Autodesk Fusion 360 part; units mm, degrees
(part 2 of 3)
sketch "Arduino" plane through (0, 0, 0) normal (0, 0, 1) x (1, 0, 0)
  line L0 (-12.271, 37.48) -> (-12.271, 41.88)
  line L1 (-4.5943, 42.08) -> (-4.7943, 41.88)
  line L2 (0, 0) -> (0, 43.18)
  line L3 (-4.7943, 42.88) -> (-4.5943, 42.68)
  line L4 (-6.271, 42.88) -> (-4.7943, 42.88)
  line L5 (-6.271, 36.18) -> (-12.271, 36.18)
  line L6 (0, 43.18) -> (-6.271, 43.18)
  line L7 (-12.271, 41.88) -> (-13.7477, 41.88)
  line L8 (-13.9477, 42.68) -> (-13.7477, 42.88)
  line L9 (-11.771, 0) -> (-6.771, 0)
  arc A0 (-4.5943, 37.28) -> (-4.5943, 36.68) centre (-4.2943, 36.98) ccw
  arc A1 (-13.9477, 42.08) -> (-13.9477, 42.68) centre (-14.2477, 42.38) ccw
  line L10 (-18.542, 43.18) -> (-18.542, 0)
  line L11 (-12.271, 36.18) -> (-12.271, 36.48)
  line L12 (-6.771, 0) -> (0, 0)
  arc A2 (-13.7477, 42.88) -> (-12.271, 42.88) centre (-13.0093, 43.6183) ccw
  arc A3 (-4.5943, 42.68) -> (-4.5943, 42.08) centre (-4.2943, 42.38) ccw
  arc A4 (-13.7477, 37.48) -> (-12.271, 37.48) centre (-13.0093, 38.2183) ccw
  arc A5 (-13.9477, 36.68) -> (-13.9477, 37.28) centre (-14.2477, 36.98) ccw
  line L13 (-18.542, 43.18) -> (0, 43.18)
  line L14 (-6.271, 41.88) -> (-6.271, 37.48)
  line L15 (-6.271, 43.18) -> (-6.271, 42.88)
  line L16 (-18.542, 0) -> (-11.771, 0)
  line L17 (-6.271, 37.48) -> (-4.7943, 37.48)
  arc A6 (-4.7943, 36.48) -> (-6.271, 36.48) centre (-5.5326, 35.7416) ccw
  line L18 (-6.271, 36.48) -> (-6.271, 36.18)
  line L19 (-4.7943, 37.48) -> (-4.5943, 37.28)
  line L20 (-4.5943, 36.68) -> (-4.7943, 36.48)
  line L21 (-13.9477, 37.28) -> (-13.7477, 37.48)
  line L22 (-13.7477, 41.88) -> (-13.9477, 42.08)
  line L23 (-12.2841, 24.6374) -> (-12.2912, 24.6445)
  line L24 (-7.771, 0.9965) -> (-6.511, 0.9965)
  circle A7 centre (-17.018, 19.156) radius 0.5
  line L25 (-12.4229, 30.5196) -> (-12.8135, 30.9102)
  circle A8 centre (-17.018, 11.656) radius 0.5
  arc A9 (-4.7943, 41.88) -> (-6.271, 41.88) centre (-5.5326, 41.1416) ccw
  circle A10 centre (-17.018, 4.156) radius 0.5
  line L26 (-8.3809, 32.7815) -> (-8.7353, 33.1359)
  line L27 (-1.524, 19.156) -> (-1.024, 19.156)
  line L28 (-5.671, 30.8528) -> (-6.0616, 30.4622)
  line L29 (-7.271, 0.2361) -> (-7.271, 1.7561)
  line L30 (-6.0786, 0) -> (-12.4635, 0)
  line L31 (-11.771, 13.9686) -> (-11.771, 18.0694)
  circle A11 centre (-17.018, 14.156) radius 0.5
  circle A12 centre (-1.524, 9.156) radius 0.5
  line L32 (-6.3515, 30.7521) -> (-5.9609, 31.1427)
  circle A13 centre (-1.524, 11.656) radius 0.5
  line L33 (-12.271, 42.88) -> (-12.271, 43.18)
  line L34 (-12.5236, 31.2001) -> (-12.133, 30.8096)
  circle A14 centre (-1.524, 19.156) radius 0.5
  circle A15 centre (-17.018, 6.656) radius 0.889
  line L35 (-6.0616, 30.4622) -> (-6.3515, 30.7521)
  arc A16 (-5.671, 31.1356) -> (-5.671, 30.8528) centre (-5.8124, 30.9942) cw
  circle A17 centre (-7.271, 3.0017) radius 0.76
  line L36 (-8.0618, 33.5265) -> (-7.9903, 33.4549)
  arc A18 (-12.0012, 24.6374) -> (-12.2841, 24.6374) centre (-12.1427, 24.7789) cw
  circle A19 centre (-17.018, 9.156) radius 0.5
  circle A20 centre (-1.524, 14.156) radius 0.5
  line L37 (-11.6107, 25.028) -> (-12.0012, 24.6374)
  line L38 (-1.524, 24.156) -> (-1.024, 24.156)
  circle A21 centre (-17.018, 9.156) radius 0.889
  line L39 (-12.4635, 4.2) -> (-6.0786, 4.2)
  line L40 (-12.271, 36.48) -> (-13.7477, 36.48)
  line L41 (-1.524, 21.656) -> (-1.024, 21.656)
  line L42 (-8.7353, 33.1359) -> (-8.3447, 33.5265)
  arc A22 (-5.9609, 31.1427) -> (-5.6781, 31.1427) centre (-5.8195, 31.0013) cw
  circle A23 centre (-1.524, 16.656) radius 0.889
  line L43 (-11.9006, 25.3179) -> (-11.6107, 25.028)
  line L44 (-7.9903, 33.1721) -> (-8.3809, 32.7815)
  line L45 (-12.271, 43.18) -> (-18.542, 43.18)
  line L46 (-12.8135, 31.1931) -> (-12.8065, 31.2001)
  arc A24 (-12.8065, 31.2001) -> (-12.5236, 31.2001) centre (-12.665, 31.0587) cw
  line L47 (-12.4635, 0) -> (-12.4635, 4.2)
  circle A25 centre (-1.524, 9.156) radius 0.889
  line L48 (-17.018, 12.156) -> (-17.018, 11.156)
  circle A26 centre (-17.018, 11.656) radius 0.889
  line L49 (-11.771, 18.0694) -> (-6.771, 18.0694)
  line L50 (-6.0786, 4.2) -> (-6.0786, 0)
  circle A27 centre (-1.524, 6.656) radius 0.889
  line L51 (0, 43.18) -> (-18.542, 43.18)
  circle A28 centre (-1.524, 16.656) radius 0.5
  circle A29 centre (-17.018, 19.156) radius 0.889
  circle A30 centre (-17.018, 14.156) radius 0.889
  line L52 (-13.7477, 36.48) -> (-13.9477, 36.68)
  circle A31 centre (-1.524, 24.156) radius 0.889
  arc A32 (-12.8135, 30.9102) -> (-12.8135, 31.1931) centre (-12.6721, 31.0517) cw
  line L53 (-12.133, 30.8096) -> (-12.4229, 30.5196)
  line L54 (-16.518, 19.156) -> (-17.018, 19.156)
  circle A33 centre (-1.524, 14.156) radius 0.889
  line L55 (-12.2912, 24.9274) -> (-11.9006, 25.3179)
  circle A34 centre (-17.018, 16.656) radius 0.889
  circle A35 centre (-1.524, 24.156) radius 0.5
  circle A36 centre (-9.271, 3) radius 0.76
  arc A37 (-7.9903, 33.4549) -> (-7.9903, 33.1721) centre (-8.1317, 33.3135) cw
  line L56 (-1.524, 39.156) -> (-1.024, 39.156)
  line L57 (-14.0003, 28.4507) -> (-9.5417, 32.9093)
  line L58 (-9.0003, 32.9093) -> (-4.5417, 28.4507)
  line L59 (-14.0589, 28.0507) -> (-14.0589, 28.3093)
  circle A38 centre (-1.524, 4.156) radius 0.889
  line L60 (-17.518, 11.656) -> (-16.518, 11.656)
  arc A39 (-6.5407, 31.7225) -> (-6.2579, 31.7225) centre (-6.3993, 31.5811) cw
  arc A40 (-6.8307, 32.2953) -> (-6.8307, 32.0124) centre (-6.9721, 32.1539) cw
  line L61 (-6.2508, 31.4326) -> (-6.6414, 31.042)
  line L62 (-6.6414, 31.042) -> (-6.9313, 31.3319)
  arc A41 (-9.5417, 32.9093) -> (-9.4003, 32.9678) centre (-9.4003, 32.7678) cw
  circle A42 centre (-17.018, 6.656) radius 0.5
  line L63 (-4.5417, 27.9093) -> (-9.0003, 23.4507)
  line L64 (-9.4003, 32.9678) -> (-9.1417, 32.9678)
  line L65 (-13.0602, 26.4776) -> (-12.7703, 26.1877)
  arc A43 (-7.7004, 32.8822) -> (-7.4176, 32.8822) centre (-7.559, 32.7408) cw
  line L66 (-13.4437, 25.7971) -> (-13.4508, 25.8042)
  arc A44 (-9.0003, 23.4507) -> (-9.1417, 23.3921) centre (-9.1417, 23.5921) cw
  arc A45 (-14.0589, 28.3093) -> (-14.0003, 28.4507) centre (-13.8589, 28.3093) cw
  circle A46 centre (-1.524, 6.656) radius 0.5
  arc A47 (-6.3083, 24.8699) -> (-6.3083, 24.5871) centre (-6.4497, 24.7285) cw
  line L67 (-15.829, 4.2) -> (-2.8014, 4.2)
  line L68 (-17.518, 6.656) -> (-16.518, 6.656)
  line L69 (-6.8307, 32.0124) -> (-7.2212, 31.6218)
  arc A48 (-12.2912, 24.6445) -> (-12.2912, 24.9274) centre (-12.1497, 24.7859) cw
  circle A49 centre (-7.271, 0.9961) radius 0.76
  line L70 (-7.2212, 31.6218) -> (-7.5112, 31.9118)
  arc A50 (-4.4831, 28.0507) -> (-4.5417, 27.9093) centre (-4.6831, 28.0507) cw
  line L71 (-5.6781, 31.1427) -> (-5.671, 31.1356)
  line L72 (-6.3083, 24.5871) -> (-6.3154, 24.58)
  arc A51 (-6.3154, 24.58) -> (-6.5982, 24.58) centre (-6.4568, 24.7214) cw
  arc A52 (-14.0003, 27.9093) -> (-14.0589, 28.0507) centre (-13.8589, 28.0507) cw
  line L73 (-6.771, 18.0694) -> (-6.771, 13.9686)
  line L74 (-6.6989, 25.2605) -> (-6.3083, 24.8699)
  line L75 (-13.4508, 26.087) -> (-13.0602, 26.4776)
  arc A53 (-4.5417, 28.4507) -> (-4.4831, 28.3093) centre (-4.6831, 28.3093) cw
  line L76 (-9.5417, 23.4507) -> (-14.0003, 27.9093)
  line L77 (-7.4176, 32.8822) -> (-7.4105, 32.8751)
  line L78 (-4.4831, 28.3093) -> (-4.4831, 28.0507)
  circle A54 centre (-1.524, 39.156) radius 0.889
  line L79 (-7.8011, 32.2017) -> (-8.091, 32.4916)
  circle A55 centre (-11.2599, 1.0002) radius 0.76
  line L80 (-8.7353, 23.2241) -> (-8.4384, 23.521)
  line L81 (-6.9888, 24.9706) -> (-6.6989, 25.2605)
  line L82 (-7.5112, 31.9118) -> (-7.1206, 32.3023)
  arc A56 (-8.3447, 33.5265) -> (-8.0618, 33.5265) centre (-8.2033, 33.385) cw
  line L83 (-12.0199, 1.0002) -> (-10.4999, 1.0002)
  line L84 (-12.7703, 26.1877) -> (-13.1609, 25.7971)
  circle A57 centre (-1.524, 36.656) radius 0.5
  circle A58 centre (-1.524, 31.656) radius 0.5
  circle A59 centre (-17.018, 31.656) radius 0.889
  arc A60 (-7.4105, 32.8751) -> (-7.4105, 32.5923) centre (-7.5519, 32.7337) cw
  line L85 (-7.4105, 32.5923) -> (-7.8011, 32.2017)
  circle A61 centre (-1.524, 4.156) radius 0.5
  line L86 (-6.2579, 31.7225) -> (-6.2508, 31.7154)
  line L87 (-1.524, 36.656) -> (-1.024, 36.656)
  line L88 (-6.771, 13.9686) -> (-11.771, 13.9686)
  arc A62 (-7.1206, 32.3023) -> (-6.8377, 32.3023) centre (-6.9791, 32.1609) cw
  arc A63 (-9.4003, 23.3921) -> (-9.5417, 23.4507) centre (-9.4003, 23.5921) cw
  line L89 (-9.1417, 23.3921) -> (-9.4003, 23.3921)
  line L90 (-6.5982, 24.58) -> (-6.9888, 24.9706)
  circle A64 centre (-17.018, 16.656) radius 0.5
  line L91 (-6.9313, 31.3319) -> (-6.5407, 31.7225)
  circle A65 centre (-17.018, 34.156) radius 0.889
  line L92 (-7.5686, 24.3907) -> (-7.2787, 24.6807)
  line L93 (-4.9019, 29.3025) -> (-5.1918, 29.5924)
  line L94 (-8.0478, 22.8476) -> (-8.0618, 22.8335)
  line L95 (-1.524, 29.156) -> (-1.024, 29.156)
  circle A66 centre (-1.524, 36.656) radius 0.889
  line L96 (-6.0184, 25.1598) -> (-6.409, 25.5504)
  line L97 (-5.1486, 25.7467) -> (-5.1557, 25.7396)
  line L98 (-4.5688, 26.3265) -> (-4.5759, 26.3195)
  arc A67 (-3.996, 26.8993) -> (-4.2789, 26.8993) centre (-4.1375, 27.0407) cw
  arc A68 (-6.2508, 31.7154) -> (-6.2508, 31.4326) centre (-6.3922, 31.574) cw
  line L99 (-1.524, 34.156) -> (-1.024, 34.156)
  line L100 (-5.4818, 29.8824) -> (-5.7717, 30.1723)
  arc A69 (-3.9245, 29.3891) -> (-3.9245, 29.1063) centre (-4.0659, 29.2477) cw
  line L101 (-17.018, 37.156) -> (-17.018, 36.156)
  circle A70 centre (-11.269, 3) radius 0.76
  arc A71 (-8.0478, 23.1304) -> (-8.0478, 22.8476) centre (-8.1892, 22.989) cw
  arc A72 (-5.1486, 26.0296) -> (-5.1486, 25.7467) centre (-5.2901, 25.8881) cw
  line L102 (-5.0982, 30.5629) -> (-5.0912, 30.5558)
  line L103 (-5.5392, 26.4201) -> (-5.1486, 26.0296)
  line L104 (-4.8587, 26.3195) -> (-5.2493, 26.7101)
  line L105 (-7.4679, 23.4274) -> (-7.475, 23.4203)
  line L106 (-8.4384, 23.521) -> (-8.0478, 23.1304)
  arc A73 (-4.8013, 29.983) -> (-4.5184, 29.983) centre (-4.6598, 29.8416) cw
  line L107 (-4.612, 29.0126) -> (-4.2214, 29.4032)
  line L108 (-6.8881, 24.0072) -> (-6.8952, 24.0002)
  line L109 (-5.0912, 30.2729) -> (-5.4818, 29.8824)
  line L110 (-4.2789, 26.8993) -> (-4.6695, 27.2899)
  line L111 (-7.178, 24.0002) -> (-7.5686, 24.3907)
  line L112 (-3.9245, 29.1063) -> (-4.3151, 28.7157)
  arc A74 (-5.7355, 25.1598) -> (-6.0184, 25.1598) centre (-5.8769, 25.3012) cw
  arc A75 (-5.1557, 25.7396) -> (-5.4385, 25.7396) centre (-5.2971, 25.8811) cw
  arc A76 (-5.7285, 25.4497) -> (-5.7285, 25.1669) centre (-5.8699, 25.3083) cw
  arc A77 (-5.3811, 30.5629) -> (-5.0982, 30.5629) centre (-5.2397, 30.4214) cw
  line L113 (-4.3151, 28.7157) -> (-4.612, 29.0126)
  arc A78 (-4.5759, 26.3195) -> (-4.8587, 26.3195) centre (-4.7173, 26.4609) cw
  arc A79 (-4.5688, 26.6094) -> (-4.5688, 26.3265) centre (-4.7102, 26.468) cw
  line L114 (-5.2493, 26.7101) -> (-4.9594, 27)
  line L115 (-4.3151, 27.6443) -> (-3.9245, 27.2537)
  arc A80 (-4.5113, 29.976) -> (-4.5113, 29.6931) centre (-4.6528, 29.8345) cw
  arc A81 (-13.4508, 25.8042) -> (-13.4508, 26.087) centre (-13.3094, 25.9456) cw
  line L116 (-4.6695, 27.2899) -> (-4.3151, 27.6443)
  arc A82 (-4.2214, 29.4032) -> (-3.9386, 29.4032) centre (-4.08, 29.2618) cw
  line L117 (-3.9386, 29.4032) -> (-3.9245, 29.3891)
  arc A83 (-7.4679, 23.7102) -> (-7.4679, 23.4274) centre (-7.6094, 23.5688) cw
  line L118 (-5.4385, 25.7396) -> (-5.8291, 26.1302)
  arc A84 (-13.1609, 25.7971) -> (-13.4437, 25.7971) centre (-13.3023, 25.9385) cw
  line L119 (-4.5184, 29.983) -> (-4.5113, 29.976)
  arc A85 (-5.0912, 30.5558) -> (-5.0912, 30.2729) centre (-5.2326, 30.4144) cw
  arc A86 (-6.8881, 24.2901) -> (-6.8881, 24.0072) centre (-7.0295, 24.1486) cw
  line L120 (-4.5113, 29.6931) -> (-4.9019, 29.3025)
  line L121 (-6.8377, 32.3023) -> (-6.8307, 32.2953)
  line L122 (-8.091, 32.4916) -> (-7.7004, 32.8822)
  line L123 (-5.7717, 30.1723) -> (-5.3811, 30.5629)
  arc A87 (-8.0618, 22.8335) -> (-8.3447, 22.8335) centre (-8.2033, 22.9749) cw
  arc A88 (-9.1417, 32.9678) -> (-9.0003, 32.9093) centre (-9.1417, 32.7678) cw
  line L124 (-5.1918, 29.5924) -> (-4.8013, 29.983)
  line L125 (-7.8585, 24.1008) -> (-7.4679, 23.7102)
  arc A89 (-7.475, 23.4203) -> (-7.7579, 23.4203) centre (-7.6164, 23.5618) cw
  line L126 (-6.119, 25.8403) -> (-5.7285, 25.4497)
  line L127 (-8.3447, 22.8335) -> (-8.7353, 23.2241)
  line L128 (-4.9594, 27) -> (-4.5688, 26.6094)
  line L129 (-3.9245, 26.9708) -> (-3.996, 26.8993)
  circle A90 centre (-1.524, 34.156) radius 0.5
  line L130 (-8.1484, 23.8109) -> (-7.8585, 24.1008)
  arc A91 (-11.067, 32.9396) -> (-10.7841, 32.9396) centre (-10.9256, 32.7982) cw
  line L131 (-11.364, 32.3598) -> (-10.9734, 31.9692)
  circle A92 centre (-1.524, 29.156) radius 0.5
  line L132 (-1.524, 26.656) -> (-1.024, 26.656)
  arc A93 (-3.9245, 27.2537) -> (-3.9245, 26.9708) centre (-4.0659, 27.1122) cw
  arc A94 (-12.2337, 31.4901) -> (-12.2337, 31.7729) centre (-12.0923, 31.6315) cw
  line L133 (-11.6539, 32.3527) -> (-11.6468, 32.3598)
  line L134 (-11.8431, 31.0995) -> (-12.2337, 31.4901)
  arc A95 (-14.6175, 29.1063) -> (-14.6175, 29.3891) centre (-14.4761, 29.2477) cw
  line L135 (-13.1034, 30.6203) -> (-12.7129, 30.2297)
  circle A96 centre (-1.524, 26.656) radius 0.5
  line L136 (-10.9734, 31.9692) -> (-11.2633, 31.6793)
  circle A97 centre (-17.018, 24.156) radius 0.889
  line L137 (-12.8639, 25.2173) -> (-12.871, 25.2243)
  line L138 (-12.2337, 31.7729) -> (-12.2266, 31.78)
  arc A98 (-12.2266, 31.78) -> (-11.9438, 31.78) centre (-12.0852, 31.6386) cw
  line L139 (-6.409, 25.5504) -> (-6.119, 25.8403)
  arc A99 (-11.6539, 32.0699) -> (-11.6539, 32.3527) centre (-11.5125, 32.2113) cw
  line L140 (-14.6175, 29.3891) -> (-14.5459, 29.4607)
  arc A100 (-10.4801, 33.5265) -> (-10.1973, 33.5265) centre (-10.3387, 33.385) cw
  circle A101 centre (-17.018, 29.156) radius 0.889
  line L141 (-13.3934, 30.6132) -> (-13.3863, 30.6203)
  line L142 (-13.9732, 30.0334) -> (-13.9661, 30.0405)
  arc A102 (-14.5459, 29.4607) -> (-14.2631, 29.4607) centre (-14.4045, 29.3192) cw
  line L143 (-13.6833, 30.0405) -> (-13.2927, 29.6499)
  line L144 (-14.0306, 26.6668) -> (-13.6401, 27.0574)
  line L145 (-7.7579, 23.4203) -> (-8.1484, 23.8109)
  line L146 (-7.2787, 24.6807) -> (-6.8881, 24.2901)
  line L147 (-13.2927, 29.6499) -> (-13.5826, 29.36)
  line L148 (-13.8725, 29.0701) -> (-14.2269, 28.7157)
  arc A103 (-13.3863, 30.6203) -> (-13.1034, 30.6203) centre (-13.2449, 30.4789) cw
  arc A104 (-14.6175, 26.9708) -> (-14.6175, 27.2537) centre (-14.4761, 27.1122) cw
  line L149 (-10.1973, 33.5265) -> (-9.8067, 33.1359)
  arc A105 (-12.871, 25.2243) -> (-12.871, 25.5072) centre (-12.7296, 25.3658) cw
  arc A106 (-13.9661, 30.0405) -> (-13.6833, 30.0405) centre (-13.8247, 29.8991) cw
  line L150 (-12.4804, 25.8978) -> (-12.1905, 25.6079)
  arc A107 (-12.5811, 25.2173) -> (-12.8639, 25.2173) centre (-12.7225, 25.3587) cw
  line L151 (-14.2269, 28.7157) -> (-14.6175, 29.1063)
  line L152 (-13.93, 27.3473) -> (-14.3206, 26.9568)
  line L153 (-13.3501, 26.7675) -> (-13.7407, 26.3769)
  circle A108 centre (-1.524, 26.656) radius 0.889
  line L154 (-5.8291, 26.1302) -> (-5.5392, 26.4201)
  arc A109 (-13.3934, 30.3304) -> (-13.3934, 30.6132) centre (-13.2519, 30.4718) cw
  line L155 (-12.1905, 25.6079) -> (-12.5811, 25.2173)
  line L156 (-12.871, 25.5072) -> (-12.4804, 25.8978)
  line L157 (-5.7285, 25.1669) -> (-5.7355, 25.1598)
  line L158 (-13.5826, 29.36) -> (-13.9732, 29.7506)
  line L159 (-11.5532, 31.3894) -> (-11.8431, 31.0995)
  line L160 (-14.6175, 27.2537) -> (-14.2269, 27.6443)
  line L161 (-13.6401, 27.0574) -> (-13.3501, 26.7675)
  line L162 (-11.9438, 31.78) -> (-11.5532, 31.3894)
  line L163 (-9.8067, 33.1359) -> (-10.1036, 32.839)
  arc A110 (-11.0741, 32.6497) -> (-11.0741, 32.9326) centre (-10.9326, 32.7911) cw
  line L164 (-13.0028, 29.9398) -> (-13.3934, 30.3304)
  line L165 (-14.6034, 26.9568) -> (-14.6175, 26.9708)
  arc A111 (-6.8952, 24.0002) -> (-7.178, 24.0002) centre (-7.0366, 24.1416) cw
  line L166 (-14.0236, 26.3769) -> (-14.0306, 26.384)
  arc A112 (-13.7407, 26.3769) -> (-14.0236, 26.3769) centre (-13.8822, 26.5183) cw
  circle A113 centre (-1.524, 29.156) radius 0.889
  line L167 (-11.2633, 31.6793) -> (-11.6539, 32.0699)
  line L168 (-14.2631, 29.4607) -> (-13.8725, 29.0701)
  arc A114 (-14.0306, 26.384) -> (-14.0306, 26.6668) centre (-13.8892, 26.5254) cw
  arc A115 (-14.3206, 26.9568) -> (-14.6034, 26.9568) centre (-14.462, 27.0982) cw
  line L169 (-11.0741, 32.9326) -> (-11.067, 32.9396)
  line L170 (-18.542, 0) -> (-18.542, 43.18)
  line L171 (-15.829, 4.2) -> (-15.829, 43.18)
  circle A116 centre (-17.018, 31.656) radius 0.5
  circle A117 centre (-17.018, 26.656) radius 0.5
  arc A118 (-11.4214, 24.0576) -> (-11.7043, 24.0576) centre (-11.5628, 24.199) cw
  line L172 (-10.1036, 32.839) -> (-10.4942, 33.2295)
  circle A119 centre (-17.018, 34.156) radius 0.5
  line L173 (-16.518, 29.156) -> (-17.018, 29.156)
  circle A120 centre (-1.524, 39.156) radius 0.5
  circle A121 centre (-17.018, 4.156) radius 0.889
  line L174 (-1.524, 31.656) -> (-1.024, 31.656)
  line L175 (-10.6835, 32.2591) -> (-11.0741, 32.6497)
  circle A122 centre (-17.018, 39.156) radius 0.889
  line L176 (-9.8067, 23.2241) -> (-10.1973, 22.8335)
  line L177 (-10.7409, 24.1583) -> (-10.451, 23.8684)
  circle A123 centre (-17.018, 36.656) radius 0.5
  line L178 (-11.7113, 24.3475) -> (-11.3207, 24.7381)
  arc A124 (-10.8416, 23.4778) -> (-11.1244, 23.4778) centre (-10.983, 23.6192) cw
  line L179 (-16.518, 16.656) -> (-17.018, 16.656)
  line L180 (-12.7129, 30.2297) -> (-13.0028, 29.9398)
  circle A125 centre (-1.524, 21.656) radius 0.889
  line L181 (-14.2269, 27.6443) -> (-13.93, 27.3473)
  circle A126 centre (-1.524, 34.156) radius 0.9737
  circle A127 centre (-17.018, 29.156) radius 0.5
  line L182 (-10.7841, 32.9396) -> (-10.3935, 32.549)
  circle A128 centre (-17.018, 26.656) radius 0.889
  line L183 (0, 43.18) -> (0, 0)
  line L184 (-11.3207, 24.7381) -> (-11.0308, 24.4482)
  arc A129 (-13.9732, 29.7506) -> (-13.9732, 30.0334) centre (-13.8318, 29.892) cw
  arc A130 (-10.1973, 22.8335) -> (-10.4801, 22.8335) centre (-10.3387, 22.9749) cw
  line L185 (-10.1611, 23.5785) -> (-9.8067, 23.2241)
  line L186 (-16.518, 26.656) -> (-17.018, 26.656)
  line L187 (-10.3935, 32.549) -> (-10.6835, 32.2591)
  line L188 (-10.5517, 23.1879) -> (-10.1611, 23.5785)
  circle A131 centre (-17.018, 21.656) radius 0.889
  line L189 (-2.8014, 4.2) -> (-2.8014, 43.18)
  circle A132 centre (-1.524, 31.656) radius 0.9737
  circle A133 centre (-9.271, 0.998) radius 0.76
  circle A134 centre (-1.524, 19.156) radius 0.889
  arc A135 (-11.7113, 24.0647) -> (-11.7113, 24.3475) centre (-11.5699, 24.2061) cw
  line L190 (-16.518, 21.656) -> (-17.018, 21.656)
  line L191 (-10.451, 23.8684) -> (-10.8416, 23.4778)
  line L192 (-16.518, 24.156) -> (-17.018, 24.156)
  circle A136 centre (-17.018, 21.656) radius 0.5
  line L193 (-11.7043, 24.0576) -> (-11.7113, 24.0647)
  arc A137 (-11.1315, 23.4849) -> (-11.1315, 23.7677) centre (-10.9901, 23.6263) cw
  arc A138 (-11.6468, 32.3598) -> (-11.364, 32.3598) centre (-11.5054, 32.2184) cw
  circle A139 centre (-17.018, 39.156) radius 0.5
  line L194 (-17.518, 36.656) -> (-16.518, 36.656)
  line L195 (-16.518, 14.156) -> (-17.018, 14.156)
  line L196 (-10.4942, 33.5124) -> (-10.4801, 33.5265)
  line L197 (-11.1315, 23.7677) -> (-10.7409, 24.1583)
  circle A140 centre (-1.524, 11.656) radius 0.889
  arc A141 (-10.5517, 22.905) -> (-10.5517, 23.1879) centre (-10.4103, 23.0465) cw
  circle A142 centre (-17.018, 24.156) radius 0.5
  circle A143 centre (-17.018, 36.656) radius 0.889
  line L198 (-10.4801, 22.8335) -> (-10.5517, 22.905)
  line L199 (-11.1244, 23.4778) -> (-11.1315, 23.4849)
  circle A144 centre (-1.524, 21.656) radius 0.5
  arc A145 (-10.4942, 33.2295) -> (-10.4942, 33.5124) centre (-10.3528, 33.371) cw
  line L200 (-2.024, 11.656) -> (-1.024, 11.656)
  line L201 (-11.0308, 24.4482) -> (-11.4214, 24.0576)
sketch "Cable Management" plane through (0, 0, -18) normal (0, 0, -1) x (1, 0, 0)
  circle A0 centre (-13.049, 34.0489) radius 1.55
  circle A1 centre (13.049, 34.0489) radius 1.55
  line L0 (13.049, 34.0489) -> (13.049, 26.0489) construction
  line L1 (0, 0) -> (-33.329, 14.3434) construction
  circle A2 centre (13.049, -34.7379) radius 1.55
  line L2 (13.049, 26.0489) -> (-33.1654, 26.0489) construction
  line L3 (-13.049, 34.0489) -> (-33.1654, 34.0489) construction
  line L4 (107.424, -7.4117) -> (107.424, 64.6535) construction
  line L5 (107.424, 64.6535) -> (-120.0387, 64.6535) construction
  line L6 (-120.0387, 64.6535) -> (-120.0387, -64.455) construction
  line L7 (-120.0387, -64.455) -> (-85.2001, -64.455) construction
  circle A3 centre (-107.5383, -7.4166) radius 1.55
  line L8 (-107.5383, -7.4166) -> (-107.5383, -54.8501) construction
  arc A4 (-84.3286, -41.8567) -> (-84.3286, -41.2595) centre (-82.8076, -41.5581) ccw
  line L9 (-2.4424, 27.3913) -> (-2.4424, 73.9863)
  line L10 (-89.3076, -41.5581) -> (-89.3076, -48.5863) construction
  line L11 (-89.3076, -48.5863) -> (-76.4539, -48.5863) construction
  line L12 (-76.4539, -48.5863) -> (-76.4539, 38.6391) construction
  line L13 (-76.4539, 38.6391) -> (31.271, 38.6391) construction
  line L14 (31.271, 38.6391) -> (31.271, 21.1451) construction
  line L15 (31.271, 21.1451) -> (-2.7267, 21.1451) construction
  line L16 (-2.7267, 21.1451) -> (-2.655, 15.7792) construction
  arc A5 (87.6714, -41.8567) -> (87.6714, -41.2595) centre (89.1924, -41.5581) ccw
  line L17 (-70.0576, 73.9863) -> (-70.0576, 2.155)
  line L18 (-33.1654, 34.0489) -> (-70.0576, 34.0489) construction
  line L19 (-33.1654, 26.0489) -> (-64.1025, 26.0489) construction
  line L20 (-33.329, 14.3434) -> (-58.5721, 14.3434) construction
  line L21 (-5.0576, -74) -> (4.9424, -74)
  line L22 (-0.0576, -74) -> (-0.0576, -26.7379) construction
  circle A6 centre (-0.0576, -69.99) radius 1.55
  circle A7 centre (-0.0576, -64.1328) radius 1.55
  circle A8 centre (-0.0576, -58.2757) radius 1.55
  circle A9 centre (-0.0576, -52.4185) radius 1.55
  circle A10 centre (-0.0576, -46.5614) radius 1.55
  circle A11 centre (-0.0576, -40.7043) radius 1.55
  circle A12 centre (-0.0576, -34.8471) radius 1.55
  circle A13 centre (-0.0576, -28.99) radius 1.55
  line L23 (-0.0576, -28.99) -> (13.049, -28.99) construction
  line L24 (13.049, -28.99) -> (13.049, -34.7379) construction
  line L25 (-13.1642, -34.387) -> (-0.0576, -34.8471)
  line L26 (-0.0576, -40.7043) -> (-58.5721, -40.7043) construction
  line L27 (-0.0576, -46.5614) -> (-64.1025, -46.5614) construction
  line L28 (-0.0576, -52.4185) -> (-70.0576, -52.4185) construction
  line L29 (-0.0576, -58.2757) -> (-77.6055, -58.2757) construction
  line L30 (-0.0576, -64.1328) -> (-85.2001, -64.455) construction
  line L31 (-58.5721, 14.3434) -> (-58.5721, -40.7043) construction
  line L32 (-64.1025, 26.0489) -> (-64.1025, -46.5614) construction
  line L33 (-70.0576, 34.0489) -> (-70.0576, -52.4185) construction
  line L34 (-107.5383, -54.8501) -> (-107.5383, -58.2757) construction
  line L35 (-107.5383, -58.2757) -> (-77.6055, -58.2757) construction
  line L36 (-1.6076, -28.99) -> (-1.6076, -69.99)
  arc A14 (-1.6076, -69.99) -> (1.4924, -69.99) centre (-0.0576, -69.99) ccw
  line L37 (1.4924, -69.99) -> (1.4924, -28.99)
  arc A15 (1.4924, -28.99) -> (-1.6076, -28.99) centre (-0.0576, -28.99) ccw
  line L38 (-0.0576, -28.99) -> (-0.0576, -69.99) construction
  line L39 (-0.0576, -46.5614) -> (1.4924, -46.5614) construction
  line L40 (-0.0576, -69.99) -> (-0.0576, -74)
  line L41 (90.7424, -74) -> (90.7424, -69)
  arc A16 (90.7424, -69) -> (87.6424, -69) centre (89.1924, -69) ccw
  line L42 (87.6424, -69) -> (87.6424, -74)
  arc A17 (87.6424, -74) -> (90.7424, -74) centre (89.1924, -74) ccw
  line L43 (1.4924, -74) -> (1.4924, -69.99)
  arc A18 (1.4924, -69.99) -> (-1.6076, -69.99) centre (-0.0576, -69.99) ccw
  line L44 (-1.6076, -69.99) -> (-1.6076, -74)
  arc A19 (-1.6076, -74) -> (1.4924, -74) centre (-0.0576, -74) ccw
  line L45 (-0.0576, -74) -> (-0.0576, -69.99) construction
  arc A20 (7.4924, -69.99) -> (4.3924, -69.99) centre (5.9424, -69.99) ccw
  line L46 (4.3924, -69.99) -> (4.3924, -74)
  line L47 (7.4924, -74) -> (7.4924, -69.99)
  arc A21 (4.3924, -74) -> (7.4924, -74) centre (5.9424, -74) ccw
  arc A22 (13.4924, -69.99) -> (10.3924, -69.99) centre (11.9424, -69.99) ccw
  line L48 (10.3924, -69.99) -> (10.3924, -74)
  line L49 (13.4924, -74) -> (13.4924, -69.99)
  arc A23 (10.3924, -74) -> (13.4924, -74) centre (11.9424, -74) ccw
  arc A24 (19.4924, -69.99) -> (16.3924, -69.99) centre (17.9424, -69.99) ccw
  line L50 (16.3924, -69.99) -> (16.3924, -74)
  line L51 (19.4924, -74) -> (19.4924, -69.99)
  arc A25 (16.3924, -74) -> (19.4924, -74) centre (17.9424, -74) ccw
  arc A26 (25.4924, -69.99) -> (22.3924, -69.99) centre (23.9424, -69.99) ccw
  line L52 (22.3924, -69.99) -> (22.3924, -74)
  line L53 (25.4924, -74) -> (25.4924, -69.99)
  arc A27 (22.3924, -74) -> (25.4924, -74) centre (23.9424, -74) ccw
  arc A28 (31.4924, -69.99) -> (28.3924, -69.99) centre (29.9424, -69.99) ccw
  line L54 (28.3924, -69.99) -> (28.3924, -74)
  line L55 (31.4924, -74) -> (31.4924, -69.99)
  arc A29 (28.3924, -74) -> (31.4924, -74) centre (29.9424, -74) ccw
  arc A30 (37.4924, -69.99) -> (34.3924, -69.99) centre (35.9424, -69.99) ccw
  line L56 (34.3924, -69.99) -> (34.3924, -74)
  line L57 (37.4924, -74) -> (37.4924, -69.99)
  arc A31 (34.3924, -74) -> (37.4924, -74) centre (35.9424, -74) ccw
  arc A32 (43.4924, -69.99) -> (40.3924, -69.99) centre (41.9424, -69.99) ccw
  line L58 (40.3924, -69.99) -> (40.3924, -74)
  line L59 (43.4924, -74) -> (43.4924, -69.99)
  arc A33 (40.3924, -74) -> (43.4924, -74) centre (41.9424, -74) ccw
  arc A34 (83.2424, -69) -> (80.1424, -69) centre (81.6924, -69) ccw
  line L60 (80.1424, -69) -> (80.1424, -74)
  arc A35 (80.1424, -74) -> (83.2424, -74) centre (81.6924, -74) ccw
  line L61 (83.2424, -74) -> (83.2424, -69)
  arc A36 (75.7424, -69) -> (72.6424, -69) centre (74.1924, -69) ccw
  line L62 (72.6424, -69) -> (72.6424, -74)
  arc A37 (72.6424, -74) -> (75.7424, -74) centre (74.1924, -74) ccw
  line L63 (75.7424, -74) -> (75.7424, -69)
  arc A38 (68.2424, -69) -> (65.1424, -69) centre (66.6924, -69) ccw
  line L64 (65.1424, -69) -> (65.1424, -74)
  arc A39 (65.1424, -74) -> (68.2424, -74) centre (66.6924, -74) ccw
  line L65 (68.2424, -74) -> (68.2424, -69)
  arc A40 (60.7424, -69) -> (57.6424, -69) centre (59.1924, -69) ccw
  line L66 (57.6424, -69) -> (57.6424, -74)
  arc A41 (57.6424, -74) -> (60.7424, -74) centre (59.1924, -74) ccw
  line L67 (60.7424, -74) -> (60.7424, -69)
  line L68 (81.6924, -69) -> (81.6924, -42.1581) construction
  line L69 (74.1924, -69) -> (74.1924, 52.9097) construction
  line L70 (-82.8076, 46.7769) -> (-82.8076, -41.5581) construction
  arc A42 (53.2424, -69) -> (50.1424, -69) centre (51.6924, -69) ccw
  line L71 (50.1424, -69) -> (50.1424, -74)
  arc A43 (50.1424, -74) -> (53.2424, -74) centre (51.6924, -74) ccw
  line L72 (53.2424, -74) -> (53.2424, -69)
  line L73 (-82.8076, 53.0508) -> (66.6924, 53.0508) construction
  line L74 (66.6924, 53.0508) -> (66.6924, -69) construction
  line L75 (59.1924, -69) -> (59.1924, 46.7769) construction
  line L76 (59.1924, 46.7769) -> (-82.8076, 46.7769) construction
  line L77 (51.6924, -69) -> (51.6924, 15.7697) construction
  line L78 (51.6924, 15.7697) -> (2.6428, 15.7697) construction
  line L79 (41.9424, -69.99) -> (41.9424, -34.7379) construction
  line L80 (41.9424, -34.7379) -> (13.049, -34.7379) construction
  line L81 (41.9424, -34.7379) -> (-0.0576, -69.99) construction
  line L82 (35.9424, -69.99) -> (35.9424, -39.7739) construction
  line L83 (5.9424, -69.99) -> (5.9424, -64.954) construction
  line L84 (-0.0576, -64.1328) -> (5.9424, -64.954) construction
  line L85 (11.9424, -69.99) -> (11.9424, -59.9179) construction
  line L86 (-0.0576, -58.2757) -> (11.9424, -59.9179) construction
  line L87 (17.9424, -69.99) -> (17.9424, -54.8819) construction
  line L88 (-0.0576, -52.4185) -> (17.9424, -54.8819) construction
  line L89 (23.9424, -69.99) -> (23.9424, -49.8459) construction
  line L90 (-0.0576, -46.5614) -> (23.9424, -49.8459) construction
  line L91 (29.9424, -69.99) -> (29.9424, -44.8099) construction
  line L92 (-0.0576, -40.7043) -> (11.9424, -44.0082) construction
  line L93 (11.9424, -44.0082) -> (29.9424, -44.8099) construction
  line L94 (35.9424, -39.7739) -> (13.0118, -39.7739) construction
  line L95 (13.0118, -39.7739) -> (-0.0576, -34.8471) construction
  line L96 (89.1924, -41.5581) -> (89.1924, -69) construction
  line L97 (-89.3076, -41.5581) -> (-89.3065, 53.1098) construction
  line L98 (-89.3065, 53.1098) -> (-89.3076, 60.048) construction
  line L99 (-89.3076, 60.048) -> (89.1924, 60.0769) construction
  line L100 (89.1924, 60.0769) -> (89.1924, 53.0508) construction
  line L101 (89.1924, 53.0508) -> (89.1924, -41.5581) construction
  line L102 (81.6924, -42.1581) -> (82.8412, -41.5581) construction
  point P0 (81.1845, 53.4097)
  point P1 (-0.0576, -74)
  dimension "d137" = 8
  dimension "d139" = 3.1
  dimension "d142" = 0
  dimension "d143" = 41
  dimension "d144" = 3.1
  dimension "d145" = 5
  dimension "d146" = 3.1
  dimension "d147" = 3.1
  dimension "d150" = 42
  dimension "d151" = 0
  dimension "d154" = -30
  dimension "d155" = 0
  constraint coincident A1.centre L0.start
  constraint vertical L0
  constraint coincident L1.start origin
  constraint perpendicular L0 L2
  constraint coincident A0.centre L3.start
  constraint parallel L2 L3
  constraint vertical L4
  constraint perpendicular L4 L5
  constraint perpendicular L5 L6
  constraint perpendicular L6 L7
  constraint coincident A3.centre L8.start
  constraint vertical L8
  constraint perpendicular L10 L11
  constraint perpendicular L11 L12
  constraint perpendicular L10 L13
  constraint perpendicular L11 L14
  constraint perpendicular L14 L15
  constraint coincident L17 L18.end
  constraint perpendicular L17 L18
  constraint perpendicular L18 L33
  constraint parallel L2 L19
  constraint perpendicular L2 L32
  constraint horizontal L20
  constraint perpendicular L20 L31
  constraint midpoint L21 P1
  constraint coincident L22 A6.centre
  constraint coincident A13.centre L23.start
  constraint perpendicular L22 L23
  constraint coincident A2.centre L24.end
  constraint perpendicular L23 L24
  constraint coincident A12.centre L25.end
  constraint coincident A11.centre L26.start
  constraint perpendicular L26 L31
  constraint coincident A10.centre L27.start
  constraint perpendicular L27 L32
  constraint coincident A9.centre L28.start
  constraint perpendicular L28 L33
  constraint coincident A8.centre L29.start
  constraint coincident A7.centre L30.start
  constraint perpendicular L29 L34
  constraint perpendicular L34 L35
  constraint tangent L36 A14
  constraint tangent A14 L37
  constraint parallel L36 L37
  constraint tangent L37 A15
  constraint tangent L36 A15
  constraint coincident A6.centre A14.centre
  constraint parallel L22 L38
  constraint coincident A10 L39.end
  constraint perpendicular L38 L39
  constraint coincident P1 L22.start
  constraint tangent L41 A16
  constraint tangent A16 L42
  constraint parallel L41 L42
  constraint tangent L42 A17
  constraint tangent L41 A17
  constraint tangent L43 A18
  constraint tangent A18 L44
  constraint parallel L43 L44
  constraint tangent L44 A19
  constraint tangent L43 A19
  constraint parallel L22 L45
  constraint coincident A34.centre L68.start
  constraint coincident A36.centre L69.start
  constraint coincident A4.centre L70.end
  constraint perpendicular L69 L73
  constraint coincident A38.centre L74.end
  constraint perpendicular L73 L74
  constraint coincident A40.centre L75.start
  constraint perpendicular L13 L75
  constraint perpendicular L70 L76
  constraint coincident A42.centre L77.start
  constraint perpendicular L77 L78
  constraint coincident A32.centre L79.start
  constraint parallel L24 L79
  constraint perpendicular L24 L80
  constraint coincident A30.centre L82.start
  constraint coincident L81 L82.end
  constraint parallel L57 L82
  constraint coincident A20.centre L83.start
  constraint coincident L81 L83.end
  constraint vertical L83
  constraint coincident A22.centre L85.start
  constraint coincident L81 L85.end
  constraint parallel L83 L85
  constraint coincident A24.centre L87.start
  constraint coincident L81 L87.end
  constraint parallel L85 L87
  constraint coincident A26.centre L89.start
  constraint coincident L81 L89.end
  constraint parallel L87 L89
  constraint coincident A28.centre L91.start
  constraint coincident L81 L91.end
  constraint parallel L89 L91
  constraint perpendicular L82 L94
  constraint coincident A5.centre L96.start
  constraint coincident A16.centre L96.end
  constraint perpendicular L98 L99
  constraint vertical L100
  measures "d137" distance of A1.centre L0.end
  measures "d139" diameter of A6
  measures "d144" diameter of A14
  measures "d145" distance of A17.centre A16.centre
  measures "d146" diameter of A16
  measures "d147" diameter of A18